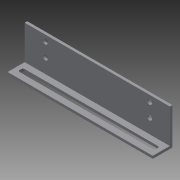
# Autodesk Inventor part: Fork 22 ver2
Saved by Autodesk Inventor 2015 (Build 190159000, 159)
## iProperties
Created: 2015-06-20
Part Number: Fork 22 ver2
Material: 一般
Document SubType Name: Modeling
Designer: kenta
Density: 1 g/cm^3
Appearance: 既定
Author: kenta
Autodesk Inventor part; units mm, degrees
ref_plane "YZ Plane" through (0, 0, 0) normal (1, 0, 0) x (0, 1, 0)
ref_plane "XZ Plane" through (0, 0, 0) normal (0, 1, 0) x (-1, 0, 0)
ref_plane "XY Plane" through (0, 0, 0) normal (0, 0, 1) x (1, 0, 0)
sketch "スケッチ1" plane through (0, 0, 0) normal (0, 0, 1) x (1, 0, 0)
  line L0 (-22.5, 88.75) -> (22.5, 88.75)
  line L1 (22.5, 88.75) -> (22.5, -88.75)
  line L2 (22.5, -88.75) -> (-22.5, -88.75)
  line L3 (-22.5, -88.75) -> (-22.5, 88.75)
  line L4 (-22.5, 88.75) -> (22.5, -88.75) construction
  line L5 (22.5, 88.75) -> (-22.5, -88.75) construction
  point P0 (0, 0)
  dimension "d0" = 45
  dimension "d1" = 177.5
  constraints: 12 end point, 2 midpoint, 2 parallel, 1 horizontal, 1 perpendicular
  measures "d0" distance of L1.end L2.end
  measures "d1" distance of L0.end L1.end
extrude "押し出し1" add sketch "スケッチ1" along normal blind 1.5
sketch "スケッチ2" plane through (0, 0, 1.5) normal (0, 0, 1) x (1, 0, 0)
  line L0 (12.5, 88.75) -> (-12.5, 88.75)
  line L1 (-12.5, 88.75) -> (-12.5, -78.75)
  line L2 (-12.5, -78.75) -> (12.5, -78.75)
  line L3 (12.5, -78.75) -> (12.5, 88.75)
  line L4 (22.5, 88.75) -> (-22.5, 88.75) projected
  point P0 (0, 0)
  dimension "d4" = 25
  dimension "d5" = 167.5
  dimension "d8" = 0
  constraints: 8 end point, 2 parallel, 1 horizontal, 1 perpendicular
  measures "d4" distance of L2.end L1.end
  measures "d5" distance of L1.end L0.end
  measures "d8" distance between parallel lines of L4 L0
extrude "押し出し2" cut sketch "スケッチ2" against normal blind 1.5
sketch "スケッチ3" plane through (0, 0, 1.5) normal (0, 0, 1) x (1, 0, 0)
  line L0 (22.5, -88.75) -> (22.5, 88.75) projected
  line L1 (-22.5, 88.75) -> (-22.5, -88.75) projected
  line L2 (22.5, 88.75) -> (12.5, 88.75) projected
  point P0 (0, 0)
  point P1 (17.5, -1.25)
  point P2 (17.5, -11.25)
  point P3 (-17.5, -1.25)
  point P4 (-17.5, -11.25)
  dimension "d9" = 5
  dimension "d10" = 5
  dimension "d11" = 90
  dimension "d12" = 10
  constraints: 2 horizontal alignment, 2 vertical alignment
  measures "d9" distance from line of point (17.5, -1.25) L0
  measures "d10" distance from line of point (-17.5, -1.25) L1
  measures "d11" distance from line of point (17.5, -1.25) L2
  measures "d12" distance of point (17.5, -11.25) point (17.5, -1.25)
hole "穴1" at (17.5, -1.25, 1.5) at (17.5, -11.25, 1.5) at (-17.5, -1.25, 1.5) at (-17.5, -11.25, 1.5) direction (0, 0, -1) diameter 3.1 depth 8 tip angle 118
sketch "スケッチ4" plane through (-22.5, -88.75, 0) normal (-1, 0, 0) x (0, 0, 1)
  line L0 (0, 0) -> (1.5, 0)
  line L1 (1.5, 0) -> (1.5, 10)
  line L2 (1.5, 10) -> (0, 10)
  line L3 (0, 10) -> (0, 0)
  point P0 (0, 88.75)
  dimension "d20" = 1.5
  dimension "d21" = 10
  constraints: 8 end point, 2 parallel, 1 horizontal, 1 perpendicular
  measures "d20" distance of L2.end L1.end
  measures "d21" distance of L1.end L0.end
extrude "押し出し3" add sketch "スケッチ4" along normal blind 20
sketch "スケッチ5" plane through (22.5, -88.75, 0) normal (1, 0, 0) x (0, 0, -1)
  line L0 (0, 0) -> (-1.5, 0)
  line L1 (-1.5, 0) -> (-1.5, 10)
  line L2 (-1.5, 10) -> (0, 10)
  line L3 (0, 10) -> (0, 0)
  point P0 (0, 88.75)
  dimension "d24" = 1.5
  dimension "d25" = 10
  constraints: 8 end point, 2 parallel, 1 horizontal, 1 perpendicular
  measures "d24" distance of L1.end L2.end
  measures "d25" distance of L0.end L1.end
extrude "押し出し4" add sketch "スケッチ5" along normal blind 20
sketch "スケッチ6" plane through (0, 0, 1.5) normal (0, 0, 1) x (1, 0, 0)
  line L0 (-40, -82.25) -> (40, -82.25)
  line L1 (40, -82.25) -> (40, -85.25)
  line L2 (40, -85.25) -> (-40, -85.25)
  line L3 (-40, -85.25) -> (-40, -82.25)
  line L4 (-40, -82.25) -> (40, -85.25) construction
  line L5 (40, -82.25) -> (-40, -85.25) construction
  line L6 (12.5, -78.75) -> (-12.5, -78.75) projected
  line L7 (42.5, -78.75) -> (42.5, -88.75) projected
  point P0 (0, 0)
  point P1 (0, -83.75)
  dimension "d28" = 80
  dimension "d29" = 3
  dimension "d30" = 3.5
  dimension "d34" = 2.5
  constraints: 12 end point, 2 midpoint, 2 parallel, 1 horizontal, 1 perpendicular
  measures "d28" distance of L1.end L2.end
  measures "d29" distance of L0.end L1.end
  measures "d30" distance between parallel lines of L0 L6
  measures "d34" distance between parallel lines of L7 L1
extrude "押し出し5" cut sketch "スケッチ6" against normal blind 20
fillet "フィレット1" radius 1 4 edges at (-40, -82.25, 0.75) (-40, -85.25, 0.75) (40, -85.25, 0.75) (40, -82.25, 0.75)
sketch "スケッチ7" plane through (0, 0, 1.5) normal (0, 0, 1) x (1, 0, 0)
  line L0 (-52.5149, -78.75) -> (41.9629, -78.75)
  line L1 (41.9629, -78.75) -> (41.9629, 114.9684)
  line L2 (41.9629, 114.9684) -> (-52.5149, 114.9684)
  line L3 (-52.5149, 114.9684) -> (-52.5149, -78.75)
  line L4 (22.5, -78.75) -> (42.5, -78.75) projected
  point P0 (0, 0)
  dimension "d35" = 0
  constraints: 8 end point, 2 parallel, 1 horizontal, 1 perpendicular
  measures "d35" distance between parallel lines of L4 L0
extrude "押し出し6" cut sketch "スケッチ7" against normal blind 10
sketch "スケッチ8" plane through (-42.5, -78.75, 1.5) normal (0, 1, 0) x (1, 0, 0)
  line L0 (0, -20) -> (85, -20)
  line L1 (85, -20) -> (85, 1.5)
  line L2 (85, 1.5) -> (0, 1.5)
  line L3 (0, 1.5) -> (0, -20)
  line L4 (0, 0) -> (0, 1.5) projected
  line L5 (0, 1.5) -> (85, 1.5) projected
  point P0 (42.5, 1.5)
  dimension "d38" = 85
  dimension "d39" = 21.5
  dimension "d40" = 0
  dimension "d41" = 0
  constraints: 8 end point, 2 parallel, 1 horizontal, 1 perpendicular
  measures "d38" distance of L2.end L1.end
  measures "d39" distance of L1.end L0.end
  measures "d40" distance between parallel lines of L4 L3
  measures "d41" distance between parallel lines of L5 L2
extrude "押し出し7" add sketch "スケッチ8" along normal blind 1.5
sketch "スケッチ10" plane through (-42.5, -77.25, 1.5) normal (0, 1, 0) x (1, 0, 0)
  line L0 (0, -20) -> (85, -20) projected
  line L1 (0, 1.5) -> (0, -20) projected
  point P0 (42.5, 1.5)
  point P1 (12, -16.5)
  point P2 (12, -8.5)
  point P3 (73, -16.5)
  point P4 (73, -8.5)
  dimension "d51" = 3.5
  dimension "d52" = 8
  dimension "d54" = 3.5
  dimension "d55" = 30.5
  dimension "d56" = 30.5
  constraints: 2 horizontal alignment, 2 vertical alignment
  measures "d51" distance from line of point (73, -16.5) L0
  measures "d52" distance of point (73, -16.5) point (73, -8.5)
  measures "d54" distance from line of point (12, -16.5) L0
  measures "d55" horizontal distance of point (73, -8.5) point (42.5, 1.5)
  measures "d56" horizontal distance of point (12, -8.5) point (42.5, 1.5)
hole "穴2" at (-30.5, -77.25, 18) at (-30.5, -77.25, 10) at (30.5, -77.25, 18) at (30.5, -77.25, 10) direction (0, -1, 0) diameter 3.1 end through all
